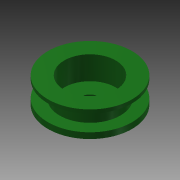
# Autodesk Inventor part: Belt Tensioner
Saved by Autodesk Inventor 2015 SP1 (Build 190203100, 203)
## iProperties
Created: 2015-02-24
Part Number: Belt Tensioner
Material: PC/ABS Plastic
Document SubType Name: Modeling
Designer: Andrew
Density: 0.357273 g/cm^3
Appearance: Smooth - Dark Forest Green
Author: Andrew
Autodesk Inventor part; units mm, degrees
ref_plane "YZ Plane" through (0, 0, 0) normal (1, 0, 0) x (0, 1, 0)
ref_plane "XZ Plane" through (0, 0, 0) normal (0, 1, 0) x (-1, 0, 0)
ref_plane "XY Plane" through (0, 0, 0) normal (0, 0, 1) x (1, 0, 0)
sketch "Sketch1" plane through (0, 0, 0) normal (0, 0, 1) x (1, 0, 0)
  circle A0 centre (0, 0) radius 11
  circle A1 centre (0, 0) radius 18
  circle A2 centre (0, 0) radius 13
  dimension "d0" = 22
  dimension "d2" = 2
  dimension "d3" = 5
  constraints: 3 centre point, 3 coincident
  measures "d0" diameter of A0
  measures "d2" radial gap between concentric circles of A0 A2
  measures "d3" radial gap between concentric circles of A2 A1
extrude "Extrusion1" add sketch "Sketch1" along normal mid plane 10 contours A1 | A2
extrude "Extrusion2" cut sketch "Sketch1" along normal mid plane 7 contours A1
sketch "Sketch2" plane through (0, 0, -5) normal (0, 0, -1) x (-1, 0, 0)
  circle A0 centre (0, 0) radius 4
  circle A1 centre (0, 0) radius 18 projected
  dimension "d8" = 8
  constraints: 1 centre point, 1 coincident
  measures "d8" diameter of A0
extrude "Extrusion3" add sketch "Sketch2" along normal blind 1
body "Solid1"
